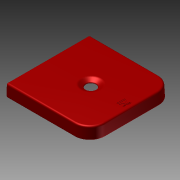
# Autodesk Inventor part: Shaft Encoder Top
Saved by Autodesk Inventor 2013 (Build 170138000, 138)
## iProperties
Created: 2012-04-06
Part Number: Shaft Encoder Top
Document SubType Name: Modeling
Designer: Phillip
Density: 1 g/cm^3
Material: Generic
Author: Phillip
Autodesk Inventor part; units mm, degrees
ref_plane "YZ Plane" through (0, 0, 0) normal (1, 0, 0) x (0, 1, 0)
ref_plane "XZ Plane" through (0, 0, 0) normal (0, 1, 0) x (-1, 0, 0)
ref_plane "XY Plane" through (0, 0, 0) normal (0, 0, 1) x (1, 0, 0)
ref_plane "Work Plane1" through (22.0547, -24.3051, 6.891) normal (-0.0000058, 0, 1) x (1, 0, 0.0000058)
ref_plane "Work Plane2" through (-0.2413, -0.0003, 0) normal (0, 0, 1) x (1, 0.0000444, 0)
sketch "Sketch2" plane through (-0.2413, -0.0003, 0) normal (0, 0, 1) x (1, 0.0000444, 0)
  line L0 (-24.8337, 16.0587) -> (-24.8227, 16.0587) projected
  arc A0 (-18.0016, 22.5035) -> (-24.8227, 16.0587) centre (-18.0016, 15.6714) ccw projected
  line L1 (-18.0016, 22.5035) -> (22.0569, 22.5035) projected
  line L2 (22.0569, 22.5035) -> (22.0569, 24.5461) projected
  line L3 (22.0569, 24.5461) -> (-17.8902, 24.5461) projected
  ellipse E0 centre (-17.8792, 15.549) end of major axis (-24.2449, 21.915) minor radius 8.9916 (-17.8902, 24.5461) -> (-26.8763, 15.5604) ccw projected
  line L4 (-26.8777, -15.5591) -> (-26.8763, 15.5604) projected
  ellipse E1 centre (-17.8806, -15.5485) end of major axis (-24.2465, -21.9141) minor radius 8.9916 (-26.8777, -15.5591) -> (-17.8916, -24.5456) ccw projected
  line L5 (22.0569, -24.5456) -> (-17.8916, -24.5456) projected
  line L6 (22.0569, -24.5456) -> (22.0569, -22.5085) projected
  line L7 (22.0569, -22.5085) -> (-18.0016, -22.5085) projected
  arc A1 (-24.8227, -16.0636) -> (-18.0016, -22.5085) centre (-18.0016, -15.6764) ccw projected
  line L8 (-24.8227, -16.0636) -> (-24.8337, -16.0636) projected
  line L9 (-24.8337, -16.0636) -> (-24.8337, -9.9768) projected
  line L10 (-24.8337, -9.9768) -> (-24.8337, 9.9718) projected
  line L11 (-24.8337, 9.9718) -> (-24.8337, 16.0587) projected
  line L12 (22.0569, -24.5456) -> (-26.8777, -24.5456)
  line L13 (-26.8777, -24.5456) -> (-26.8777, 24.5461)
  line L14 (-26.8777, 24.5461) -> (22.0569, 24.5461)
  line L15 (22.0569, -22.5085) -> (-24.8337, -22.5085)
  line L16 (-24.8337, -22.5085) -> (-24.8337, 22.5035)
  line L17 (-24.8337, 22.5035) -> (22.0569, 22.5035)
  line L18 (22.0569, -22.5085) -> (22.0569, 22.5035)
  point P0 (0.2413, 0.0003)
  constraints: 14 end point, 3 perpendicular, 2 collinear, 2 point on line, 2 other
ref_plane "Work Plane3" through (21.8145, -24.3043, 6.891) normal (-0.0000058, 0, 1) x (1, 0.0000444, 0.0000058)
extrude "Extrusion3" add sketch "Sketch2" along normal up to surface (6.8909 mm away)
ref_plane "Work Plane4" through (-18.2456, -22.5096, 6.8908) normal (-0.0000058, 0, 1) x (1, 0.0000444, 0.0000058)
draft "FaceDraft3" angle 2 pull direction (0, 0, 1) faces at (5.503, 24.5461, 2.297) (-27.1194, 8.1807, 2.297) (-10.8064, -24.5464, 2.297) fixed edges at (-2.6528, 24.5457, 0) (-27.119, -0.0012, 0) (-2.6506, -24.546, 0)
fillet "Fillet5" radius 8.9916 2 edges at (-26.9998, 24.4243, 3.4454) (-26.9976, -24.4268, 3.4454)
shell "Shell1" thickness 1.8034 removed faces 2 at (8.4998, -8.1816, 0) at (21.8159, -8.1008, 2.297)
sketch "Sketch4" plane through (-0.2413, -0.0003, 0) normal (0, 0, -1) x (-1, -0.0000444, 0)
  line L0 (25.0732, 15.5578) -> (25.0732, -15.5573) projected
  ellipse E0 centre (17.8806, -15.5485) end of major axis (22.9696, -20.6375) minor radius 7.1882 (17.8894, -22.7411) -> (25.0732, -15.5573) ccw projected
  line L1 (25.0732, -15.2945) -> (23.2698, -15.2945)
  line L2 (23.2698, -15.2945) -> (23.2698, -9.7827)
  line L3 (23.2698, -9.7827) -> (25.0732, -9.7827)
  line L4 (25.0732, -9.7827) -> (25.0732, -15.2945)
  point P0 (-0.2413, 0.0003)
  dimension "d15" = 0.254
  dimension "d16" = 5.5118
  dimension "d17" = 1.8034
  constraints: 8 end point, 2 parallel, 1 collinear, 1 horizontal, 1 perpendicular, 1 other
  measures "d15" distance from line of L1 point (17.881, -15.549)
  measures "d16" distance of L1.end L2.end
  measures "d17" distance of L2.end L3.end
extrude "Extrusion4" add sketch "Sketch4" against normal up to next
fillet "Fillet6" radius 0.508 2 edges at (-23.5107, -9.784, 2.5437) (-23.5104, -15.2958, 2.5437)
ref_plane "Work Plane5" through (21.8156, 0.001, 5.0876) normal (-0.0000444, 1, 0) x (-1, -0.0000444, 0)
mirror "Mirror1" about plane through (21.8156, 0.001, 5.0876) normal (-0.0000444, 1, 0) of "Extrusion4", "Fillet6"
sketch "Sketch6" plane through (21.8167, -24.3043, 6.891) normal (-0.0000058, 0, 1) x (1, 0.0000444, 0.0000058)
  circle A0 centre (-24.9787, 24.3005) radius 3.7464 projected
  circle A1 centre (-24.9787, 24.3005) radius 2.9972
  point P0 (-21.8156, 24.3052)
  dimension "d24" = 5.9944
  constraints: 1 centre point, 1 coincident
  measures "d24" diameter of A1
hole "Hole1" at (-3.1631, -0.0049, 6.8908) direction (0.0000058, 0, -1) diameter 5.9944 depth 3.175 tip angle 118 countersink diameter 10.9982 countersink angle 120
fillet "Fillet7" radius 0.508 1 edges at (-3.1631, 2.9923, 5.4464)
fillet "Fillet8" radius 2.0066 1 edges at (-3.1631, 5.4942, 6.8908)
fillet "Fillet9" radius 0.9906 5 edges at (1.9606, 24.3053, 6.8909) (-24.248, 21.6728, 6.8909) (-26.8784, -0.0012, 6.8909) (-24.2461, -21.675, 6.8909) (1.9627, -24.3052, 6.8909)
fillet "Fillet10" radius 0.9906 2 edges at (21.8166, -23.6427, 0) (21.8145, 23.6446, 0)
fillet "Fillet11" radius 0.508 12 edges at (1.3471, -24.5458, 0) (21.5265, -24.5348, 0.2901) (21.8167, -24.424, 3.4627) (21.8166, -24.0358, 6.6128) (21.8156, 0.001, 6.8909) (21.8145, 24.0377, 6.6128) (21.8145, 24.4259, 3.4627) (21.5243, 24.5367, 0.2901) (1.3449, 24.5459, 0) (-24.4887, 21.9135, 0) (-27.119, -0.0012, 0) (-24.4867, -21.9157, 0)
sketch "Sketch7" plane through (-25.9211, -15.3537, 6.8907) normal (-0.0000058, 0, 1) x (1, 0.0000444, 0.0000058)
  line L0 (0, 0) -> (0, 30.705) projected
  line L1 (2.8268, 15.3437) -> (4.1258, 13.0937)
  line L2 (4.1258, 13.0937) -> (4.1258, 17.5937)
  line L3 (4.1258, 17.5937) -> (2.8268, 15.3437)
  line L4 (2.1353, 16.8396) -> (2.1779, 16.9126)
  line L5 (2.1779, 16.9126) -> (2.1991, 17.0099)
  line L6 (2.1991, 17.0099) -> (2.1991, 17.2045)
  line L7 (2.1991, 17.2045) -> (2.1779, 17.3018)
  line L8 (2.1779, 17.3018) -> (2.1353, 17.3747)
  line L9 (2.1353, 17.3747) -> (2.0715, 17.4234)
  line L10 (2.0715, 17.4234) -> (1.9864, 17.4477)
  line L11 (1.9864, 17.4477) -> (1.6672, 17.4477)
  line L12 (1.6672, 17.4477) -> (1.5821, 17.4234)
  line L13 (1.5821, 17.4234) -> (1.5183, 17.3747)
  line L14 (1.5183, 17.3747) -> (1.4757, 17.3018)
  line L15 (1.4757, 17.3018) -> (1.4545, 17.2045)
  line L16 (1.4545, 17.2045) -> (1.4545, 17.0099)
  line L17 (1.4545, 17.0099) -> (1.4757, 16.9126)
  line L18 (1.4757, 16.9126) -> (1.5183, 16.8396)
  line L19 (1.5183, 16.8396) -> (1.5821, 16.791)
  line L20 (1.5821, 16.791) -> (1.6672, 16.7666)
  line L21 (1.6672, 16.7666) -> (1.9864, 16.7666)
  line L22 (1.9864, 16.7666) -> (2.0715, 16.791)
  line L23 (2.0715, 16.791) -> (2.1353, 16.8396)
  line L24 (2.2204, 15.818) -> (2.2204, 16.2801)
  line L25 (2.2204, 16.2801) -> (1.9013, 16.2801)
  line L26 (1.9013, 16.2801) -> (1.9013, 15.818)
  line L27 (1.9013, 15.818) -> (1.9225, 15.745)
  line L28 (1.9225, 15.745) -> (1.9651, 15.6964)
  line L29 (1.9651, 15.6964) -> (2.0289, 15.672)
  line L30 (2.0289, 15.672) -> (2.0928, 15.672)
  line L31 (2.0928, 15.672) -> (2.1566, 15.6964)
  line L32 (2.1566, 15.6964) -> (2.1991, 15.745)
  line L33 (2.1991, 15.745) -> (2.2204, 15.818)
  line L34 (2.3055, 17.3261) -> (2.3268, 17.2045)
  line L35 (2.3268, 17.2045) -> (2.3268, 17.0099)
  line L36 (2.3268, 17.0099) -> (2.3055, 16.8883)
  line L37 (2.3055, 16.8883) -> (2.263, 16.791)
  line L38 (2.263, 16.791) -> (2.1779, 16.6937)
  line L39 (2.1779, 16.6937) -> (2.0928, 16.645)
  line L40 (2.0928, 16.645) -> (1.9864, 16.6207)
  line L41 (1.9864, 16.6207) -> (1.6672, 16.6207)
  line L42 (1.6672, 16.6207) -> (1.5608, 16.645)
  line L43 (1.5608, 16.645) -> (1.4757, 16.6937)
  line L44 (1.4757, 16.6937) -> (1.3906, 16.791)
  line L45 (1.3906, 16.791) -> (1.3481, 16.8883)
  line L46 (1.3481, 16.8883) -> (1.3268, 17.0099)
  line L47 (1.3268, 17.0099) -> (1.3268, 17.2045)
  line L48 (1.3268, 17.2045) -> (1.3481, 17.3261)
  line L49 (1.3481, 17.3261) -> (1.3906, 17.4234)
  line L50 (1.3906, 17.4234) -> (1.4757, 17.5207)
  line L51 (1.4757, 17.5207) -> (1.5608, 17.5693)
  line L52 (1.5608, 17.5693) -> (1.6672, 17.5937)
  line L53 (1.6672, 17.5937) -> (1.9864, 17.5937)
  line L54 (1.9864, 17.5937) -> (2.0928, 17.5693)
  line L55 (2.0928, 17.5693) -> (2.1779, 17.5207)
  line L56 (2.1779, 17.5207) -> (2.263, 17.4234)
  line L57 (2.263, 17.4234) -> (2.3055, 17.3261)
  line L58 (2.1566, 15.5504) -> (2.0928, 15.5261)
  line L59 (2.0928, 15.5261) -> (2.0076, 15.5261)
  line L60 (2.0076, 15.5261) -> (1.9438, 15.5504)
  line L61 (1.9438, 15.5504) -> (1.8587, 15.6234)
  line L62 (1.8587, 15.6234) -> (1.7949, 15.7207)
  line L63 (1.7949, 15.7207) -> (1.7736, 15.8423)
  line L64 (1.7736, 15.8423) -> (1.7736, 16.2801)
  line L65 (1.7736, 16.2801) -> (1.3268, 16.2801)
  line L66 (1.3268, 16.2801) -> (1.3268, 16.4261)
  line L67 (1.3268, 16.4261) -> (2.3268, 16.4261)
  line L68 (2.3268, 16.4261) -> (2.3268, 15.8423)
  line L69 (2.3268, 15.8423) -> (2.3055, 15.7207)
  line L70 (2.3055, 15.7207) -> (2.2417, 15.6234)
  line L71 (2.2417, 15.6234) -> (2.1566, 15.5504)
  line L72 (1.4545, 15.1856) -> (1.4545, 14.4558)
  line L73 (1.4545, 14.4558) -> (1.3268, 14.4558)
  line L74 (1.3268, 14.4558) -> (1.3268, 15.3315)
  line L75 (1.3268, 15.3315) -> (2.3268, 15.3315)
  line L76 (2.3268, 15.3315) -> (2.3268, 14.4558)
  line L77 (2.3268, 14.4558) -> (2.1991, 14.4558)
  line L78 (2.1991, 14.4558) -> (2.1991, 15.1856)
  line L79 (2.1991, 15.1856) -> (1.9225, 15.1856)
  line L80 (1.9225, 15.1856) -> (1.9225, 14.5531)
  line L81 (1.9225, 14.5531) -> (1.7949, 14.5531)
  line L82 (1.7949, 14.5531) -> (1.7949, 15.1856)
  line L83 (1.7949, 15.1856) -> (1.4545, 15.1856)
  line L84 (2.1991, 14.1153) -> (1.3268, 14.1153)
  line L85 (1.3268, 14.1153) -> (1.3268, 14.2612)
  line L86 (1.3268, 14.2612) -> (2.3268, 14.2612)
  line L87 (2.3268, 14.2612) -> (2.3268, 14.0423)
  line L88 (2.3268, 14.0423) -> (1.4757, 13.4342)
  line L89 (1.4757, 13.4342) -> (2.3268, 13.4342)
  line L90 (2.3268, 13.4342) -> (2.3268, 13.2883)
  line L91 (2.3268, 13.2883) -> (1.3268, 13.2883)
  line L92 (1.3268, 13.2883) -> (1.3268, 13.5072)
  line L93 (1.3268, 13.5072) -> (2.1991, 14.1153)
  line L94 (4.1258, 13.0937) -> (2.8268, 15.3437)
  line L95 (2.8268, 15.3437) -> (4.1258, 17.5937)
  line L96 (4.1258, 17.5937) -> (4.1258, 13.0937)
  line L97 (4.8258, 17.5937) -> (4.8258, 13.0937)
  line L98 (4.8258, 13.0937) -> (4.6258, 13.0937)
  line L99 (4.6258, 13.0937) -> (4.6258, 17.5937)
  line L100 (4.6258, 17.5937) -> (4.8258, 17.5937)
  line L101 (5.5258, 13.0937) -> (5.3258, 13.0937)
  line L102 (5.3258, 13.0937) -> (5.3258, 17.5937)
  line L103 (5.3258, 17.5937) -> (5.5258, 17.5937)
  line L104 (5.5258, 17.5937) -> (5.5258, 13.0937)
  line L105 (0, 15.3525) -> (12.6665, 15.3525) construction
  point P0 (25.9217, 15.3525)
  constraints: 210 end point, 1 midpoint, 1 parallel
emboss "Emboss1" sketch "Sketch7" operation add depth 0.2032 direction (0.0000058, 0, -1)
body "Solid3"
